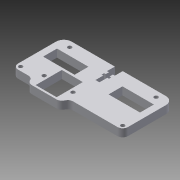
# Autodesk Inventor part: XcrLeft_a
Saved by Autodesk Inventor 2013 (Build 170138000, 138)
## iProperties
Created: 2015-01-14
Part Number: XcrLeft_a
Material: Generic
Document SubType Name: Modeling
Designer: dzban
Density: 1 g/cm^3
Author: dzban
Autodesk Inventor part; units mm, degrees
ref_plane "YZ Plane" through (0, 0, 0) normal (1, 0, 0) x (0, 1, 0)
ref_plane "XZ Plane" through (0, 0, 0) normal (0, 1, 0) x (-1, 0, 0)
ref_plane "XY Plane" through (0, 0, 0) normal (0, 0, 1) x (1, 0, 0)
sketch "Sketch1" plane through (0, 0, 0) normal (0, 0, 1) x (1, 0, 0)
  arc A0 (-78, 39) -> (-84, 33) centre (-78, 33) ccw
  line L0 (-84, 33) -> (-84, 4)
  arc A1 (-84, 4) -> (-80, 0) centre (-80, 4) ccw
  line L1 (-80, 0) -> (-72, 0)
  arc A2 (-68.2919, -2.5) -> (-72, 0) centre (-72, -4) ccw
  arc A3 (-68.2919, -2.5) -> (-64.5838, -5) centre (-64.5838, -1) ccw
  line L2 (-64.5838, -5) -> (-45.4162, -5)
  arc A4 (-45.4162, -5) -> (-41.7081, -2.5) centre (-45.4162, -1) ccw
  arc A5 (-38, 0) -> (-41.7081, -2.5) centre (-38, -4) ccw
  line L3 (-38, 0) -> (-4, 0)
  arc A6 (-4, 0) -> (0, 4) centre (-4, 4) ccw
  line L4 (0, 4) -> (0, 33)
  arc A7 (0, 33) -> (-6, 39) centre (-6, 33) ccw
  line L5 (-6, 39) -> (-39, 39)
  line L6 (-39, 39) -> (-39, 33)
  line L7 (-39, 33) -> (-40.5, 33)
  line L8 (-40.5, 33) -> (-40.5, 30.5)
  line L9 (-40.5, 30.5) -> (-39.25, 30.5)
  line L10 (-39.25, 30.5) -> (-39.25, 28.7)
  line L11 (-39.25, 28.7) -> (-40.5, 28.7)
  line L12 (-40.5, 28.7) -> (-40.5, 22.7)
  line L13 (-40.5, 22.7) -> (-43.5, 22.7)
  line L14 (-43.5, 22.7) -> (-43.5, 28.7)
  line L15 (-43.5, 28.7) -> (-44.75, 28.7)
  line L16 (-44.75, 28.7) -> (-44.75, 30.5)
  line L17 (-44.75, 30.5) -> (-43.5, 30.5)
  line L18 (-43.5, 30.5) -> (-43.5, 33)
  line L19 (-43.5, 33) -> (-45, 33)
  line L20 (-45, 33) -> (-45, 39)
  line L21 (-45, 39) -> (-78, 39)
  line L22 (-63, -3.5) -> (-63, 16.5)
  line L23 (-63, 16.5) -> (-47, 16.5)
  line L24 (-47, 16.5) -> (-47, -3.5)
  line L25 (-47, -3.5) -> (-63, -3.5)
  line L26 (-79, 18.2) -> (-79, 28.8)
  line L27 (-79, 28.8) -> (-55, 28.8)
  line L28 (-55, 28.8) -> (-55, 18.2)
  line L29 (-55, 18.2) -> (-79, 18.2)
  line L30 (-29, 18.2) -> (-29, 28.8)
  line L31 (-29, 28.8) -> (-5, 28.8)
  line L32 (-5, 28.8) -> (-5, 18.2)
  line L33 (-5, 18.2) -> (-29, 18.2)
  circle A8 centre (-66, 6) radius 1.5
  circle A9 centre (-44, 6) radius 1.5
  circle A10 centre (-3, 3) radius 1.5
  circle A11 centre (-81, 3) radius 1.5
  circle A12 centre (-75, 34.5) radius 1.5
  circle A13 centre (-9, 34.5) radius 1.5
  point P0 (0, 0)
  point P1 (0, 0)
  constraints: 68 end point, 16 point on circle, 14 centre point
extrude "Extrusion1" add sketch "Sketch1" along normal blind 6
body "Solid1"
